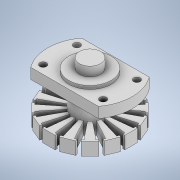
# Autodesk Inventor part: burshless_20_base
Saved by Autodesk Inventor 2020 (Build 240168000, 168)
## iProperties
Created: 2020-08-02
Part Number: burshless_20_base
Material: Generic
Document SubType Name: Modeling
Designer: psrobotics
Density: 1 g/cm^3
Appearance: Default
Author: psrobotics
Autodesk Inventor part; units mm, degrees
ref_plane "YZ Plane" through (0, 0, 0) normal (1, 0, 0) x (0, 1, 0)
ref_plane "XZ Plane" through (0, 0, 0) normal (0, 1, 0) x (-1, 0, 0)
ref_plane "XY Plane" through (0, 0, 0) normal (0, 0, 1) x (1, 0, 0)
sketch "Sketch1" plane through (0, 0, 0) normal (0, 1, 0) x (-1, 0, 0)
  circle A0 centre (0, 0) radius 10
  line L0 (11, 6) -> (11, -6)
  line L1 (11, -6) -> (-11, -6)
  line L2 (-11, -6) -> (-11, 6)
  line L3 (-11, 6) -> (11, 6)
  line L4 (11, 6) -> (-11, -6) construction
  line L5 (11, -6) -> (-11, 6) construction
  point P0 (8, 6)
  point P1 (-8, 6)
  point P2 (-8, -6)
  point P3 (8, -6)
  dimension "d0" = 20
  dimension "d1" = 12
  dimension "d2" = 22
  constraints: 12 end point, 2 midpoint, 2 parallel, 1 centre point, 1 coincident, 1 perpendicular, 1 vertical
  measures "d0" diameter of A0
  measures "d1" distance of L0.start L0.end
  measures "d2" distance of L0.end L1.end
extrude "Extrusion1" add sketch "Sketch1" along normal blind 2.5 contours A0 L1 L3
sketch "Sketch2" plane through (0, 2.5, 0) normal (0, 1, 0) x (1, 0, 0)
  circle A0 centre (0, 0) radius 5
  dimension "d5" = 10
  constraints: 1 centre point, 1 coincident
  measures "d5" diameter of A0
extrude "Extrusion2" add sketch "Sketch2" along normal blind 0.8
sketch "Sketch3" plane through (0, 2.5, 0) normal (0, 1, 0) x (1, 0, 0)
  circle A0 centre (0, 0) radius 2.5
  dimension "d8" = 5
  constraints: 1 centre point, 1 coincident
  measures "d8" diameter of A0
extrude "Extrusion3" add sketch "Sketch3" along normal blind 3
sketch "Sketch4" plane through (0, 0, 0) normal (0, -1, 0) x (1, 0, 0)
  circle A0 centre (0, 0) radius 3.85
  dimension "d11" = 7.7
  constraints: 1 centre point, 1 coincident
  measures "d11" diameter of A0
extrude "Extrusion4" add sketch "Sketch4" along normal blind 4.8
sketch "Sketch5" plane through (0, 2.5, 0) normal (0, 1, 0) x (1, 0, 0)
  line L0 (-7.1, -4) -> (-7.1, 4)
  line L1 (-7.1, 4) -> (7.1, 4)
  line L2 (7.1, 4) -> (7.1, -4)
  line L3 (7.1, -4) -> (-7.1, -4)
  line L4 (-7.1, -4) -> (7.1, 4) construction
  line L5 (-7.1, 4) -> (7.1, -4) construction
  point P0 (0, 0)
  dimension "d14" = 8
  dimension "d15" = 14.2
  constraints: 12 end point, 2 midpoint, 2 parallel, 1 perpendicular, 1 vertical
  measures "d14" distance of L0.start L0.end
  measures "d15" distance of L0.end L1.end
hole "Hole1" at (-7.1, 2.5, 4) at (-7.1, 2.5, -4) at (7.1, 2.5, 4) at (7.1, 2.5, -4) direction (0, -1, 0) diameter 1.6 depth 17
sketch "Sketch6" plane through (0, -4.8, 0) normal (0, -1, 0) x (1, 0, 0)
  circle A0 centre (0, 0) radius 2.5 projected
  line L0 (0, 0) -> (-9.5, 0)
  line L1 (-9.75, -1.5) -> (-9.25, -1.5)
  line L2 (-9.25, -1.5) -> (-9.25, 1.5)
  line L3 (-9.25, 1.5) -> (-9.75, 1.5)
  line L4 (-9.75, 1.5) -> (-9.75, -1.5)
  line L5 (-9.75, -1.5) -> (-9.25, 1.5) construction
  line L6 (-9.25, -1.5) -> (-9.75, 1.5) construction
  circle A1 centre (0, 0) radius 3.85 projected
  line L7 (-9.25, 1.5) -> (-9.25, 1)
  line L8 (-9.25, 1) -> (0, 0)
  line L9 (-9.25, -1.5) -> (-9.25, -1)
  line L10 (-9.25, -1) -> (0, 0)
  point P0 (-3.8277, 0.4138)
  point P1 (-3.8277, -0.4138)
  dimension "d23" = 9.5
  dimension "d24" = 0.5
  dimension "d25" = 3
  dimension "d26" = 0.5
  dimension "d27" = 0.5
  constraints: 22 end point, 2 midpoint, 2 parallel, 2 perpendicular, 2 point on line, 1 horizontal
  measures "d23" distance of L0.start L0.end
  measures "d24" distance of L1.start L1.end
  measures "d25" distance of L2.end L1.end
  measures "d26" distance of L2.end L7.end
  measures "d27" distance of L1.end L9.end
extrude "Extrusion5" add sketch "Sketch6" along normal blind 3 contours A1 L0 L2 L8 | L10 L2 L0 A1 | L2 L1 L4 L3
sketch "Sketch7" plane through (0, -4.8, 0) normal (0, -1, 0) x (1, 0, 0)
  arc A0 (-3.8277, -0.4138) -> (-3.8277, 0.4138) centre (0, 0) ccw projected
  arc A1 (-3.8277, 0.4138) -> (-3.8277, -0.4138) centre (0, 0) ccw projected
extrude "Extrusion6" add sketch "Sketch7" along normal blind 3
pattern_circular "Circular Pattern1" count 16 over 360 about axis through (0, 0, 0) along (0, -1, 0) of "Extrusion5"
sketch "Sketch8" plane through (0, -7.8, 0) normal (0, -1, 0) x (1, 0, 0)
  circle A0 centre (0, 0) radius 1.75
  dimension "d35" = 3.5
  constraints: 1 centre point, 1 coincident
  measures "d35" diameter of A0
extrude "Extrusion7" cut sketch "Sketch8" against normal blind 5
body "Solid1"
